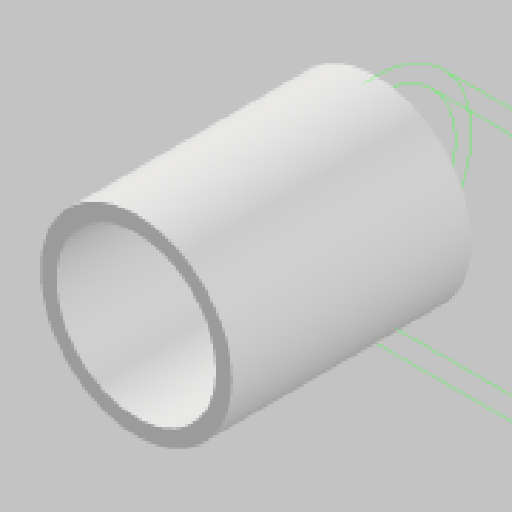
# Autodesk Inventor part: Buje azul
Saved by Autodesk Inventor 2024 (Build 280153000, 153)
## iProperties
Created: 2023-09-27
Part Number: Buje azul
Material: Generic
Document SubType Name: Modeling
Designer: ARViau
Density: 1 g/cm^3
Appearance: Default
Author: ARViau
Autodesk Inventor part; units mm, degrees
ref_plane "YZ Plane" through (0, 0, 0) normal (1, 0, 0) x (0, 1, 0)
ref_plane "XZ Plane" through (0, 0, 0) normal (0, 1, 0) x (-1, 0, 0)
ref_plane "XY Plane" through (0, 0, 0) normal (0, 0, 1) x (1, 0, 0)
sketch "Sketch1" plane through (0, 0, 0) normal (0, 0, 1) x (1, 0, 0)
  circle A0 centre (0, 0) radius 6.35 projected
  line L0 (5.08, 8.7988) -> (-5.08, 8.7988) projected
  line L1 (-5.08, 8.7988) -> (-10.16, 0) projected
  line L2 (-10.16, 0) -> (-5.08, -8.7988) projected
  line L3 (-5.08, -8.7988) -> (5.08, -8.7988) projected
  line L4 (5.08, -8.7988) -> (10.16, 0) projected
  line L5 (10.16, 0) -> (5.08, 8.7988) projected
  circle A1 centre (0, 0) radius 7.62
  dimension "d0" = 15.24
  constraints: 1 centre point, 1 coincident
  measures "d0" diameter of A1
extrude "Extrusion1" add sketch "Sketch1" along normal blind 19.05 contours A1
body "Solid1"
